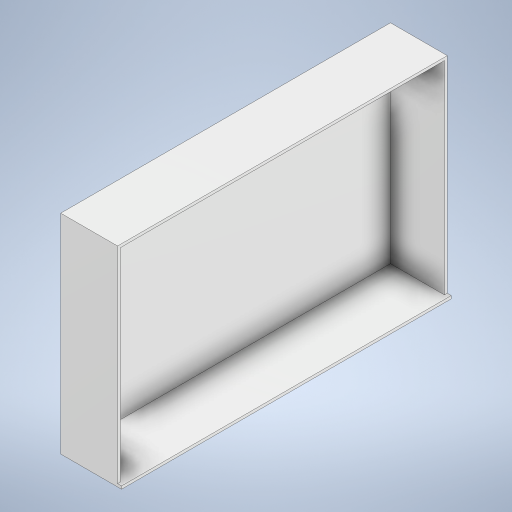
# Autodesk Inventor part: monitor_case
Saved by Autodesk Inventor 2023 (Build 270158000, 158)
## iProperties
Created: 2024-02-13
Part Number: monitor_case
Material: ABS 플라스틱
Document SubType Name: Modeling
Designer: ps737
Mass: 1030.11 g
Surface Area: 4075.8 cm^2
Volume: 971.8 cm^3
Density: 1.06 g/cm^3
Appearance: 매끄러움 - 흰색
Author: ps737
Autodesk Inventor part; units mm, degrees
ref_plane "YZ Plane" through (0, 0, 0) normal (1, 0, 0) x (0, 1, 0)
ref_plane "XZ Plane" through (0, 0, 0) normal (0, 1, 0) x (-1, 0, 0)
ref_plane "XY Plane" through (0, 0, 0) normal (0, 0, 1) x (1, 0, 0)
sketch "스케치1" plane through (0, 0, 0) normal (1, 0, 0) x (0, 1, 0)
  line L0 (367, 290) -> (0, 290)
  line L1 (0, 290) -> (0, -290)
  line L2 (0, -290) -> (367, -290)
  line L3 (367, -290) -> (367, 290)
  line L4 (362, 285) -> (5, 285)
  line L5 (5, 290) -> (5, -290)
  line L6 (5, -285) -> (362, -285)
  line L7 (362, -285) -> (362, 285)
  point P0 (0, 0)
  point P1 (0, 0)
  dimension "d0" = 367
  dimension "d1" = 580
  dimension "d2" = 5
  constraints: 16 end point, 4 parallel, 4 point on line, 2 perpendicular, 1 coincident, 1 horizontal, 1 midpoint, 1 other
  measures "d0" distance of L2.end L1.end
  measures "d1" distance of L1.end L0.end
  measures "d2" distance between parallel lines of L3 L7
extrude "돌출1" add sketch "스케치1" along normal blind 100 contours L3 L2 L5 L6 L7 L4 L0
extrude "돌출2" add sketch "스케치1" along normal blind 107 contours L5 L2 L1 L0
extrude "돌출3" add sketch "스케치1" along normal blind 5 contours L4 L7 L6 L5
